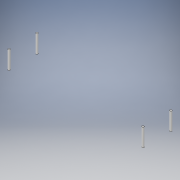
# Autodesk Inventor part: Register
Saved by Autodesk Inventor 2019 (Build 230136000, 136)
## iProperties
Created: 2020-11-05
Part Number: Register
Material: Generic
Document SubType Name: Modeling
Designer: james
Density: 1 g/cm^3
Appearance: Default
Author: james
Autodesk Inventor part; units mm, degrees
ref_plane "YZ Plane" through (0, 0, 0) normal (1, 0, 0) x (0, 1, 0)
ref_plane "XZ Plane" through (0, 0, 0) normal (0, 1, 0) x (-1, 0, 0)
ref_plane "XY Plane" through (0, 0, 0) normal (0, 0, 1) x (1, 0, 0)
sketch "Sketch1" plane through (0, 0, 0) normal (0, 1, 0) x (-1, 0, 0)
  line L0 (0, 0.0005) -> (200, -0.0005)
  line L1 (200, 0) -> (200, 48)
  line L2 (200, 48) -> (0, 48)
  line L3 (0, 48) -> (0, 0)
  circle A0 centre (4, 4) radius 0.06
  circle A1 centre (196, 44) radius 0.06
  circle A2 centre (196, 4) radius 0.06
  circle A3 centre (4, 44) radius 0.06
  circle A4 centre (4, 44) radius 1.5
  circle A5 centre (4, 4) radius 1.5
  circle A6 centre (196, 4) radius 1.5
  circle A7 centre (196, 44) radius 1.5
  arc A8 (4, 3.9192) -> (4, 4.0808) centre (4, 4) ccw
  arc A9 (4, 4.0808) -> (4, 3.9192) centre (4, 4) ccw
  arc A10 (4, 44.0808) -> (4, 43.9192) centre (4, 44) ccw
  arc A11 (196, 3.9192) -> (196, 4.0808) centre (196, 4) ccw
  arc A12 (196, 43.9192) -> (196, 44.0808) centre (196, 44) ccw
  arc A13 (196, 44.0808) -> (196, 43.9192) centre (196, 44) ccw
  arc A14 (196, 4.0808) -> (196, 3.9192) centre (196, 4) ccw
  arc A15 (4, 43.9192) -> (4, 44.0808) centre (4, 44) ccw
  arc A16 (4, 43.1992) -> (4, 44.8008) centre (4, 44) ccw
  arc A17 (4, 44.8008) -> (4, 43.1992) centre (4, 44) ccw
  arc A18 (4, 3.1992) -> (4, 4.8008) centre (4, 4) ccw
  arc A19 (4, 4.8008) -> (4, 3.1992) centre (4, 4) ccw
  arc A20 (196, 3.1992) -> (196, 4.8008) centre (196, 4) ccw
  arc A21 (196, 4.8008) -> (196, 3.1992) centre (196, 4) ccw
  arc A22 (196, 43.1992) -> (196, 44.8008) centre (196, 44) ccw
  arc A23 (196, 44.8008) -> (196, 43.1992) centre (196, 44) ccw
  arc A24 (4, 44.8008) -> (4, 43.1992) centre (4, 44) ccw
  arc A25 (196, 44.0808) -> (196, 43.9192) centre (196, 44) ccw
  arc A26 (4, 43.9192) -> (4, 44.0808) centre (4, 44) ccw
  arc A27 (4, 44.0808) -> (4, 43.9192) centre (4, 44) ccw
  arc A28 (4, 3.1992) -> (4, 4.8008) centre (4, 4) ccw
  arc A29 (4, 4.8008) -> (4, 3.1992) centre (4, 4) ccw
  arc A30 (196, 3.9192) -> (196, 4.0808) centre (196, 4) ccw
  arc A31 (196, 4.0808) -> (196, 3.9192) centre (196, 4) ccw
  arc A32 (4, 3.9192) -> (4, 4.0808) centre (4, 4) ccw
  arc A33 (196, 3.1992) -> (196, 4.8008) centre (196, 4) ccw
  arc A34 (196, 4.8008) -> (196, 3.1992) centre (196, 4) ccw
  arc A35 (4, 4.0808) -> (4, 3.9192) centre (4, 4) ccw
  arc A36 (196, 43.9192) -> (196, 44.0808) centre (196, 44) ccw
  arc A37 (4, 43.1992) -> (4, 44.8008) centre (4, 44) ccw
  arc A38 (196, 43.1992) -> (196, 44.8008) centre (196, 44) ccw
  arc A39 (196, 44.8008) -> (196, 43.1992) centre (196, 44) ccw
  line L4 (0, 0) -> (0, 48)
  line L5 (200, 48) -> (0, 48)
  line L6 (200.0051, 48) -> (200, -0.0009)
  line L7 (200, -0.0009) -> (0, 0)
  constraints: 64 point on circle, 40 centre point, 16 end point, 3 equal length, 1 point on line
extrude "Extrusion1" add sketch "Sketch1" along normal blind 25.4 contours A4 | A5 | A6 | A7 | A9 A8 | A15 A10 | A14 A11 | A13 A12 | A17 A16 | A19 A18 | A21 A20 | A23 A22
body "Solid1"
